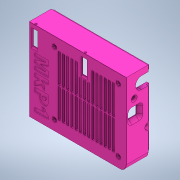
# Autodesk Inventor part: Rambo Case P1.0
Saved by Autodesk Inventor 2020.3 (Build 243373010, 373A)
## iProperties
Created: 2019-12-21
Part Number: Rambo Case P1.0
Material: Generic
Document SubType Name: Modeling
Designer: pepd9
Density: 1 g/cm^3
Appearance: Default
Author: pepd9
Autodesk Inventor part; units mm, degrees
(part 1 of 2)
ref_plane "YZ Plane" through (0, 0, 0) normal (1, 0, 0) x (0, 1, 0)
ref_plane "XZ Plane" through (0, 0, 0) normal (0, 1, 0) x (-1, 0, 0)
ref_plane "Work Plane1" through (0, 0, 3) normal (0, 0, 1) x (1, 0, 0)
sketch "Sketch1" plane through (0, 0, 3) normal (0, 0, 1) x (1, 0, 0)
  circle A0 centre (48.26, 47.625) radius 1.5 construction
  circle A1 centre (48.26, -47.625) radius 1.5 construction
  circle A2 centre (-48.26, -47.625) radius 1.5 construction
  circle A3 centre (-48.26, 47.625) radius 1.5 construction
  line L0 (60.26, 61.625) -> (-86.26, 61.625)
  line L1 (-86.26, 61.625) -> (-86.26, -62.625)
  line L2 (-86.26, -62.625) -> (60.26, -62.625)
  line L3 (60.26, -62.625) -> (60.26, 61.625)
  point P0 (0, 0)
  dimension "d1" = 14
  dimension "d2" = 12
  dimension "d3" = 38
  dimension "d4" = 15
  constraints: 8 end point, 2 parallel, 1 horizontal, 1 perpendicular
  measures "d1" distance from line of L0 A0.centre
  measures "d2" distance from line of L3 A0.centre
  measures "d3" distance from line of L1 A3.centre
  measures "d4" distance from line of L2 A1.centre
extrude "Extrusion1" add sketch "Sketch1" along normal blind 3
sketch "Sketch2" plane through (0, 0, 3) normal (0, 0, -1) x (-1, 0, 0)
  line L0 (-60.26, -62.625) -> (-60.26, 61.625) projected
  line L1 (86.26, -62.625) -> (-60.26, -62.625) projected
  line L2 (86.26, 61.625) -> (86.26, -62.625) projected
  line L3 (-60.26, 61.625) -> (86.26, 61.625) projected
  line L4 (-60.26, -62.625) -> (-60.26, 61.625) projected
  line L5 (86.26, -62.625) -> (-60.26, -62.625) projected
  line L6 (-60.26, 61.625) -> (-54.26, 61.625)
  line L7 (-54.26, 61.625) -> (-54.26, -62.625)
  line L8 (-54.26, -62.625) -> (-60.26, -62.625)
  line L9 (-60.26, -62.625) -> (-60.26, 61.625)
  line L10 (-54.26, -62.625) -> (86.26, -62.625)
  line L11 (86.26, -62.625) -> (86.26, -56.625)
  line L12 (86.26, -56.625) -> (-54.26, -56.625)
  line L13 (-54.26, -56.625) -> (-54.26, -62.625)
  line L14 (86.26, 61.625) -> (86.26, -62.625) projected
  line L15 (-54.26, 61.625) -> (86.26, 61.625)
  line L16 (86.26, 61.625) -> (86.26, 55.625)
  line L17 (86.26, 55.625) -> (-54.26, 55.625)
  line L18 (-54.26, 55.625) -> (-54.26, 61.625)
  point P0 (0, 0)
  dimension "d7" = 6
  dimension "d10" = 6
  dimension "d11" = 6
  constraints: 24 end point, 6 parallel, 3 horizontal, 3 perpendicular, 3 point on line
  measures "d7" distance of L7.end L8.end
  measures "d10" distance of L11.end L10.end
  measures "d11" distance of L15.end L16.end
extrude "Extrusion2" add sketch "Sketch2" along normal blind 30 contours L0 L3 L7 L1 | L7 L12 L2 L1 | L3 L2 L17 L7
sketch "Sketch3" plane through (0, 0, 3) normal (0, 0, -1) x (-1, 0, 0)
  circle A0 centre (-48.26, -47.625) radius 1.5 construction
  circle A1 centre (-48.26, 47.625) radius 1.5 construction
  circle A2 centre (48.26, -47.625) radius 1.5 construction
  circle A3 centre (48.26, 47.625) radius 1.5 construction
  line L0 (-52.26, -45.3156) -> (-48.26, -43.0062)
  line L1 (-48.26, -43.0062) -> (-44.26, -45.3156)
  line L2 (-44.26, -45.3156) -> (-44.26, -49.9344)
  line L3 (-44.26, -49.9344) -> (-48.26, -52.2438)
  line L4 (-48.26, -52.2438) -> (-52.26, -49.9344)
  line L5 (-52.26, -49.9344) -> (-52.26, -45.3156)
  line L6 (-52.26, 49.9344) -> (-48.26, 52.2438)
  line L7 (-48.26, 52.2438) -> (-44.26, 49.9344)
  line L8 (-44.26, 49.9344) -> (-44.26, 45.3156)
  line L9 (-44.26, 45.3156) -> (-48.26, 43.0062)
  line L10 (-48.26, 43.0062) -> (-52.26, 45.3156)
  line L11 (-52.26, 45.3156) -> (-52.26, 49.9344)
  line L12 (44.26, 49.9344) -> (48.26, 52.2438)
  line L13 (48.26, 52.2438) -> (52.26, 49.9344)
  line L14 (52.26, 49.9344) -> (52.26, 45.3156)
  line L15 (52.26, 45.3156) -> (48.26, 43.0062)
  line L16 (48.26, 43.0062) -> (44.26, 45.3156)
  line L17 (44.26, 45.3156) -> (44.26, 49.9344)
  line L18 (44.26, -45.3156) -> (48.26, -43.0062)
  line L19 (48.26, -43.0062) -> (52.26, -45.3156)
  line L20 (52.26, -45.3156) -> (52.26, -49.9344)
  line L21 (52.26, -49.9344) -> (48.26, -52.2438)
  line L22 (48.26, -52.2438) -> (44.26, -49.9344)
  line L23 (44.26, -49.9344) -> (44.26, -45.3156)
  point P0 (0, 0)
  point P1 (44.26, -47.625)
  dimension "d12" = 8
  dimension "d13" = 8
  dimension "d14" = 8
  dimension "d15" = 8
  constraints: 48 end point, 4 coincident, 3 vertical, 1 midpoint, 1 point on line, 52 other
  measures "d12" distance between parallel lines of L20 L23
  measures "d13" distance between parallel lines of L17 L14
  measures "d14" distance between parallel lines of L8 L11
  measures "d15" distance between parallel lines of L5 L2
extrude "Extrusion3" add sketch "Sketch3" along normal blind 4
sketch "Sketch4" plane through (0, 0, -1) normal (0, 0, -1) x (-1, 0, 0)
  circle A0 centre (-48.26, -47.625) radius 1.5 projected
  circle A1 centre (-48.26, 47.625) radius 1.5 projected
  circle A2 centre (48.26, 47.625) radius 1.5 projected
  circle A3 centre (48.26, -47.625) radius 1.5 projected
  point P0 (0, 0)
hole "Hole1" at (48.26, -47.625, -1) at (48.26, 47.625, -1) at (-48.26, 47.625, -1) at (-48.26, -47.625, -1) direction (0, 0, 1) diameter 3.2 end through all clearance for "Socket Head Cap Screw" size "M3" standard "Ansi Metric M Profile"
sketch "Sketch5" plane through (60.26, -62.625, 6) normal (1, 0, 0) x (0, 0, -1)
  arc A0 (8.5, 75.51) -> (8, 75.01) centre (8.5, 75.01) ccw projected
  line L0 (8.5, 75.51) -> (18.7, 75.51) projected
  arc A1 (19.2, 75.01) -> (18.7, 75.51) centre (18.7, 75.01) ccw projected
  line L1 (19.2, 64.21) -> (19.2, 75.01) projected
  arc A2 (18.7, 63.71) -> (19.2, 64.21) centre (18.7, 64.21) ccw projected
  line L2 (8.5, 63.71) -> (18.7, 63.71) projected
  arc A3 (8, 64.21) -> (8.5, 63.71) centre (8.5, 64.21) ccw projected
  line L3 (8, 75.01) -> (8, 64.21) projected
  arc A4 (7.4, 64.21) -> (8.5, 63.11) centre (8.5, 64.21) ccw
  line L4 (8.5, 63.11) -> (18.7, 63.11)
  arc A5 (18.7, 63.11) -> (19.8, 64.21) centre (18.7, 64.21) ccw
  line L5 (19.8, 64.21) -> (19.8, 75.01)
  arc A6 (19.8, 75.01) -> (18.7, 76.11) centre (18.7, 75.01) ccw
  line L6 (18.7, 76.11) -> (8.5, 76.11)
  arc A7 (8.5, 76.11) -> (7.4, 75.01) centre (8.5, 75.01) ccw
  line L7 (7.4, 75.01) -> (7.4, 64.21)
  point P0 (6, 62.625)
  dimension "d25" = 0.6
  constraints: 8 end point, 8 point on circle, 4 centre point, 7 other
  measures "d25" distance between parallel lines of L3 L7
extrude "Extrusion4" cut sketch "Sketch5" against normal up to surface (6 mm away) contours L0 A1 L1 A2 L2 A3 L3 A0 | L7 A7 L6 A6 L5 A5 L4 A4
sketch "Sketch6" plane through (60.26, -62.625, 6) normal (1, 0, 0) x (0, 0, -1)
  circle A0 centre (12, 90.819) radius 1.27
  line L0 (0, 0) -> (0, 124.25) projected
  point P0 (6, 62.625)
  dimension "d106" = 2.54
  dimension "d107" = 12
  constraints: 1 centre point
  measures "d106" diameter of A0
  measures "d107" distance from line of L0 A0.centre
hole "Hole2" at (60.26, 28.194, -6) direction (-1, 0, 0) diameter 5 end through all
chamfer "Chamfer2" distance 2 angle 45 1 edges at (60.26, 28.194, -3.5)
sketch "Sketch7" plane through (-86.26, 55.625, 3) normal (0, -1, 0) x (1, 0, 0)
  circle A0 centre (82.9724, 1) radius 1.1 projected
  circle A1 centre (8.1724, 1) radius 1.1 projected
  circle A2 centre (8.1724, 1) radius 1.1 projected
  point P0 (86.26, -3)
hole "Hole3" at (-3.2876, 55.625, 4) at (-78.0876, 55.625, 4) direction (0, 1, 0) diameter 3.2 end through all clearance for "Socket Head Cap Screw" size "M3" standard "Ansi Metric M Profile"
sketch "Sketch8" plane through (-86.26, 55.625, -27) normal (0, -1, 0) x (1, 0, 0)
  arc A0 (81.7234, 30) -> (84.2214, 30) centre (82.9724, 31) ccw projected
  arc A1 (6.9234, 30) -> (9.4214, 30) centre (8.1724, 31) ccw projected
  point P0 (86.26, 27)
  point P1 (5.1724, 31)
hole "Hole4" at (-3.2876, 55.625, 4) at (-78.0876, 55.625, 4) direction (0, -1, 0) diameter 10 depth 25
sketch "Sketch9" plane through (0, 0, 6) normal (0, 0, 1) x (1, 0, 0)
  line L0 (1.295, 55.625) -> (1.295, 30.625) projected
  line L1 (1.295, 30.625) -> (-7.8702, 30.625) projected
  line L2 (-7.8702, 30.625) -> (-7.8702, 55.625) projected
  line L3 (-7.8702, 55.625) -> (1.295, 55.625) projected
  line L4 (-73.505, 55.625) -> (-73.505, 30.625) projected
  line L5 (-73.505, 30.625) -> (-82.6702, 30.625) projected
  line L6 (-82.6702, 30.625) -> (-82.6702, 55.625) projected
  line L7 (-82.6702, 55.625) -> (-73.505, 55.625) projected
  circle A0 centre (-48.26, 47.625) radius 1.6 projected
  circle A1 centre (48.26, -47.625) radius 1.6 projected
  circle A2 centre (48.26, 47.625) radius 1.6 projected
  circle A3 centre (-48.26, -47.625) radius 1.6 projected
  line L8 (60.26, 61.625) -> (-86.26, 61.625) projected
  line L9 (-86.26, 61.625) -> (-86.26, -62.625) projected
  line L10 (-86.26, -62.625) -> (60.26, -62.625) projected
  line L11 (60.26, -62.625) -> (60.26, 61.625) projected
  line L12 (51.01, 46.0373) -> (48.26, 44.4496)
  line L13 (48.26, 44.4496) -> (45.51, 46.0373)
  line L14 (45.51, 46.0373) -> (45.51, 49.2127)
  line L15 (45.51, 49.2127) -> (48.26, 50.8004)
  line L16 (48.26, 50.8004) -> (51.01, 49.2127)
  line L17 (51.01, 49.2127) -> (51.01, 46.0373)
  line L18 (51.01, -49.2127) -> (48.26, -50.8004)
  line L19 (48.26, -50.8004) -> (45.51, -49.2127)
  line L20 (45.51, -49.2127) -> (45.51, -46.0373)
  line L21 (45.51, -46.0373) -> (48.26, -44.4496)
  line L22 (48.26, -44.4496) -> (51.01, -46.0373)
  line L23 (51.01, -46.0373) -> (51.01, -49.2127)
  circle A4 centre (-48.26, -47.625) radius 1.6 projected
  line L24 (-45.51, -49.2127) -> (-48.26, -50.8004)
  line L25 (-48.26, -50.8004) -> (-51.01, -49.2127)
  line L26 (-51.01, -49.2127) -> (-51.01, -46.0373)
  line L27 (-51.01, -46.0373) -> (-48.26, -44.4496)
  line L28 (-48.26, -44.4496) -> (-45.51, -46.0373)
  line L29 (-45.51, -46.0373) -> (-45.51, -49.2127)
  line L30 (-45.51, 46.0373) -> (-48.26, 44.4496)
  line L31 (-48.26, 44.4496) -> (-51.01, 46.0373)
  line L32 (-51.01, 46.0373) -> (-51.01, 49.2127)
  line L33 (-51.01, 49.2127) -> (-48.26, 50.8004)
  line L34 (-48.26, 50.8004) -> (-45.51, 49.2127)
  line L35 (-45.51, 49.2127) -> (-45.51, 46.0373)
  point P0 (0, 0)
  point P1 (-45.51, 47.625)
  dimension "d55" = 5.5
  dimension "d56" = 5.5
  dimension "d57" = 5.5
  constraints: 48 end point, 4 coincident, 4 vertical, 1 midpoint, 1 point on line, 52 other
  measures "d55" distance between parallel lines of L17 L14
  measures "d56" distance between parallel lines of L20 L23
  measures "d57" distance between parallel lines of L26 L29
extrude "Extrusion5" cut sketch "Sketch9" against normal blind 3 contours L12 L13 L14 L15 L16 L17 | L18 L19 L20 L21 L22 L23 | L24 L25 L26 L27 L28 L29 | L30 L31 L32 L33 L34 L35
sketch "Sketch10" plane through (0, 0, 6) normal (0, 0, 1) x (1, 0, 0)
  line L0 (-4, 45.0147) -> (-1, 45.0147)
  line L1 (-1, 45.0147) -> (-1, -44.9853)
  line L2 (-1, -44.9853) -> (-4, -44.9853)
  line L3 (-4, -44.9853) -> (-4, 45.0147)
  line L4 (-4, 45.0147) -> (-1, -44.9853) construction
  line L5 (-1, 45.0147) -> (-4, -44.9853) construction
  line L6 (45.51, -46.0373) -> (48.26, -44.4496) projected
  line L7 (48.26, -44.4496) -> (51.01, -46.0373) projected
  line L8 (51.01, -46.0373) -> (51.01, -49.2127) projected
  line L9 (51.01, -49.2127) -> (48.26, -50.8004) projected
  line L10 (48.26, -50.8004) -> (45.51, -49.2127) projected
  line L11 (45.51, -49.2127) -> (45.51, -46.0373) projected
  line L12 (-48.26, -50.8004) -> (-51.01, -49.2127) projected
  line L13 (-51.01, -49.2127) -> (-51.01, -46.0373) projected
  line L14 (-51.01, -46.0373) -> (-48.26, -44.4496) projected
  line L15 (-48.26, -44.4496) -> (-45.51, -46.0373) projected
  line L16 (-45.51, -46.0373) -> (-45.51, -49.2127) projected
  line L17 (-45.51, -49.2127) -> (-48.26, -50.8004) projected
  line L18 (48.26, 44.4496) -> (45.51, 46.0373) projected
  line L19 (45.51, 46.0373) -> (45.51, 49.2127) projected
  line L20 (45.51, 49.2127) -> (48.26, 50.8004) projected
  line L21 (48.26, 50.8004) -> (51.01, 49.2127) projected
  line L22 (51.01, 49.2127) -> (51.01, 46.0373) projected
  line L23 (51.01, 46.0373) -> (48.26, 44.4496) projected
  line L24 (-45.51, 49.2127) -> (-45.51, 46.0373) projected
  line L25 (-45.51, 46.0373) -> (-48.26, 44.4496) projected
  line L26 (-48.26, 44.4496) -> (-51.01, 46.0373) projected
  line L27 (-51.01, 46.0373) -> (-51.01, 49.2127) projected
  line L28 (-51.01, 49.2127) -> (-48.26, 50.8004) projected
  line L29 (-48.26, 50.8004) -> (-45.51, 49.2127) projected
  line L30 (1.295, 55.625) -> (1.295, 30.625) projected
  line L31 (1.295, 30.625) -> (-7.8702, 30.625) projected
  line L32 (-7.8702, 30.625) -> (-7.8702, 55.625) projected
  line L33 (-7.8702, 55.625) -> (1.295, 55.625) projected
  line L34 (-73.505, 55.625) -> (-73.505, 30.625) projected
  line L35 (-73.505, 30.625) -> (-82.6702, 30.625) projected
  line L36 (-82.6702, 30.625) -> (-82.6702, 55.625) projected
  line L37 (-82.6702, 55.625) -> (-73.505, 55.625) projected
  line L38 (60.26, 61.625) -> (-86.26, 61.625) projected
  line L39 (-86.26, 61.625) -> (-86.26, -62.625) projected
  line L40 (-86.26, -62.625) -> (60.26, -62.625) projected
  line L41 (60.26, -62.625) -> (60.26, 61.625) projected
  line L42 (5.295, 26.625) -> (5.295, 59.625)
  line L43 (5.295, 59.625) -> (-11.8702, 59.625)
  line L44 (-11.8702, 59.625) -> (-11.8702, 26.625)
  line L45 (-11.8702, 26.625) -> (5.295, 26.625)
  line L46 (2.2, 45.0147) -> (5.2, 45.0147)
  line L47 (2.2, -44.9853) -> (2.2, 45.0147)
  line L48 (5.2, 45.0147) -> (5.2, -44.9853)
  line L49 (5.2, -44.9853) -> (2.2, -44.9853)
  line L50 (8.4, 45.0147) -> (11.4, 45.0147)
  line L51 (8.4, -44.9853) -> (8.4, 45.0147)
  line L52 (11.4, 45.0147) -> (11.4, -44.9853)
  line L53 (11.4, -44.9853) -> (8.4, -44.9853)
  line L54 (14.6, 45.0147) -> (17.6, 45.0147)
  line L55 (14.6, -44.9853) -> (14.6, 45.0147)
  line L56 (17.6, 45.0147) -> (17.6, -44.9853)
  line L57 (17.6, -44.9853) -> (14.6, -44.9853)
  line L58 (20.8, 45.0147) -> (23.8, 45.0147)
  line L59 (20.8, -44.9853) -> (20.8, 45.0147)
  line L60 (23.8, 45.0147) -> (23.8, -44.9853)
  line L61 (23.8, -44.9853) -> (20.8, -44.9853)
  line L62 (27, 45.0147) -> (30, 45.0147)
  line L63 (27, -44.9853) -> (27, 45.0147)
  line L64 (30, 45.0147) -> (30, -44.9853)
  line L65 (30, -44.9853) -> (27, -44.9853)
  line L66 (33.2, 45.0147) -> (36.2, 45.0147)
  line L67 (33.2, -44.9853) -> (33.2, 45.0147)
  line L68 (36.2, 45.0147) -> (36.2, -44.9853)
  line L69 (36.2, -44.9853) -> (33.2, -44.9853)
  line L70 (39.4, 45.0147) -> (42.4, 45.0147)
  line L71 (39.4, -44.9853) -> (39.4, 45.0147)
  line L72 (42.4, 45.0147) -> (42.4, -44.9853)
  line L73 (42.4, -44.9853) -> (39.4, -44.9853)
  line L74 (-10.4, -44.9853) -> (-10.4, 45.0147)
  line L75 (-7.4, 45.0147) -> (-7.4, -44.9853)
  line L76 (-10.4, 45.0147) -> (-7.4, 45.0147)
  line L77 (-7.4, -44.9853) -> (-10.4, -44.9853)
  line L78 (-16.8, -44.9853) -> (-16.8, 45.0147)
  line L79 (-13.8, 45.0147) -> (-13.8, -44.9853)
  line L80 (-16.8, 45.0147) -> (-13.8, 45.0147)
  line L81 (-13.8, -44.9853) -> (-16.8, -44.9853)
  line L82 (-23.2, -44.9853) -> (-23.2, 45.0147)
  line L83 (-20.2, 45.0147) -> (-20.2, -44.9853)
  line L84 (-23.2, 45.0147) -> (-20.2, 45.0147)
  line L85 (-20.2, -44.9853) -> (-23.2, -44.9853)
  line L86 (-29.6, -44.9853) -> (-29.6, 45.0147)
  line L87 (-26.6, 45.0147) -> (-26.6, -44.9853)
  line L88 (-29.6, 45.0147) -> (-26.6, 45.0147)
  line L89 (-26.6, -44.9853) -> (-29.6, -44.9853)
  line L90 (-36, -44.9853) -> (-36, 45.0147)
  line L91 (-33, 45.0147) -> (-33, -44.9853)
  line L92 (-36, 45.0147) -> (-33, 45.0147)
  line L93 (-33, -44.9853) -> (-36, -44.9853)
  line L94 (-42.4, -44.9853) -> (-42.4, 45.0147)
  line L95 (-39.4, 45.0147) -> (-39.4, -44.9853)
  line L96 (-42.4, 45.0147) -> (-39.4, 45.0147)
  line L97 (-39.4, -44.9853) -> (-42.4, -44.9853)
  point P0 (-7.4, 26.625)
  point P1 (-10.4, 26.625)
  point P2 (-1, 26.625)
  point P3 (-4, 26.625)
  point P4 (4.1765, 45.0147)
  point P5 (2.2, 26.625)
  point P6 (5.2, 26.625)
  dimension "d60" = 3
  dimension "d61" = 90
  dimension "d62" = 4
  dimension "d65" = 6.2
  dimension "d72" = 6.4
  dimension "d77" = 3.11
  dimension "d78" = 1.0226
  constraints: 124 end point, 3 horizontal, 2 collinear, 2 parallel, 1 perpendicular, 105 other
  measures "d60" distance of L1.end L2.end
  measures "d61" distance of L0.end L1.end
  measures "d62" distance between parallel lines of L30 L42
  measures "d65" distance of L0.start L46.start
  measures "d72" distance of L2.end L74.start
  measures "d77" distance between parallel lines of L19 L72
  measures "d78" distance from line of L18.end L70
extrude "Extrusion6" cut sketch "Sketch10" against normal blind 3 contours L45 L1 L2 L3 | L75 L77 L74 L45 | L45 L48 L49 L47 | L50 L52 L53 L51 | L54 L56 L57 L55 | L58 L60 L61 L59 | L62 L64 L65 L63 | L66 L68 L69 L67 | L70 L72 L73 L71 | L78 L80 L79 L81 | L82 L84 L83 L85 | L86 L88 L87 L89 | L90 L92 L91 L93 | L94 L96 L95 L97
sketch "Sketch11" plane through (0, 0, 6) normal (0, 0, 1) x (1, 0, 0)
  line L0 (45.51, -46.0373) -> (48.26, -44.4496) projected
  line L1 (48.26, -44.4496) -> (51.01, -46.0373) projected
  line L2 (51.01, -46.0373) -> (51.01, -49.2127) projected
  line L3 (51.01, -49.2127) -> (48.26, -50.8004) projected
  line L4 (48.26, -50.8004) -> (45.51, -49.2127) projected
  line L5 (45.51, -49.2127) -> (45.51, -46.0373) projected
  line L6 (-48.26, -50.8004) -> (-51.01, -49.2127) projected
  line L7 (-51.01, -49.2127) -> (-51.01, -46.0373) projected
  line L8 (-51.01, -46.0373) -> (-48.26, -44.4496) projected
  line L9 (-48.26, -44.4496) -> (-45.51, -46.0373) projected
  line L10 (-45.51, -46.0373) -> (-45.51, -49.2127) projected
  line L11 (-45.51, -49.2127) -> (-48.26, -50.8004) projected
  line L12 (48.26, 44.4496) -> (45.51, 46.0373) projected
  line L13 (45.51, 46.0373) -> (45.51, 49.2127) projected
  line L14 (45.51, 49.2127) -> (48.26, 50.8004) projected
  line L15 (48.26, 50.8004) -> (51.01, 49.2127) projected
  line L16 (51.01, 49.2127) -> (51.01, 46.0373) projected
  line L17 (51.01, 46.0373) -> (48.26, 44.4496) projected
  line L18 (-45.51, 49.2127) -> (-45.51, 46.0373) projected
  line L19 (-45.51, 46.0373) -> (-48.26, 44.4496) projected
  line L20 (-48.26, 44.4496) -> (-51.01, 46.0373) projected
  line L21 (-51.01, 46.0373) -> (-51.01, 49.2127) projected
  line L22 (-51.01, 49.2127) -> (-48.26, 50.8004) projected
  line L23 (-48.26, 50.8004) -> (-45.51, 49.2127) projected
  line L24 (1.295, 55.625) -> (1.295, 30.625) projected
  line L25 (1.295, 30.625) -> (-7.8702, 30.625) projected
  line L26 (-7.8702, 30.625) -> (-7.8702, 55.625) projected
  line L27 (-7.8702, 55.625) -> (1.295, 55.625) projected
  line L28 (-73.505, 55.625) -> (-73.505, 30.625) projected
  line L29 (-73.505, 30.625) -> (-82.6702, 30.625) projected
  line L30 (-82.6702, 30.625) -> (-82.6702, 55.625) projected
  line L31 (-82.6702, 55.625) -> (-73.505, 55.625) projected
  line L32 (60.26, 61.625) -> (-86.26, 61.625) projected
  line L33 (-86.26, 61.625) -> (-86.26, -62.625) projected
  line L34 (-86.26, -62.625) -> (60.26, -62.625) projected
  line L35 (60.26, -62.625) -> (60.26, 61.625) projected
  line L36 (-42.4, 45.0147) -> (-42.4, -44.9853) projected
  line L37 (42.4, 1.2) -> (-42.4, 1.2)
  line L38 (-42.4, 1.2) -> (-42.4, -1.2)
  line L39 (-42.4, -1.2) -> (42.4, -1.2)
  line L40 (42.4, -1.2) -> (42.4, 1.2)
  line L41 (42.4, 1.2) -> (-42.4, -1.2) construction
  line L42 (-42.4, 1.2) -> (42.4, -1.2) construction
  point P0 (0, 0)
  dimension "d81" = 2.4
  constraints: 12 end point, 2 midpoint, 2 parallel, 1 horizontal, 1 perpendicular, 1 point on line
  measures "d81" distance of L38.end L37.end
extrude "Extrusion7" add sketch "Sketch11" against normal up to surface (3 mm away) contours L37 L40 L39 L36
fillet "Fillet1" radius 0.4 50 edges at (42.4, 45.0147, 4.5) (39.4, 45.0147, 4.5) (36.2, 45.0147, 4.5) (33.2, 45.0147, 4.5) (30, 45.0147, 4.5) (27, 45.0147, 4.5) (23.8, 45.0147, 4.5) (20.8, 45.0147, 4.5) (14.6, 45.0147, 4.5) (17.6, 45.0147, 4.5) (11.4, 45.0147, 4.5) (8.4, 45.0147, 4.5) (42.4, 1.2, 4.5) (39.4, 1.2, 4.5) (39.4, -1.2, 4.5) (42.4, -1.2, 4.5) (42.4, -44.9853, 4.5) (39.4, -44.9853, 4.5) (36.2, -44.9853, 4.5) (33.2, -44.9853, 4.5) (30, -44.9853, 4.5) (27, -44.9853, 4.5) (23.8, -44.9853, 4.5) (20.8, -44.9853, 4.5) (17.6, -44.9853, 4.5) (14.6, -44.9853, 4.5) (11.4, -44.9853, 4.5) (8.4, -44.9853, 4.5) (5.2, -44.9853, 4.5) (2.2, -44.9853, 4.5) (-1, -44.9853, 4.5) (-4, -44.9853, 4.5) (-7.4, -44.9853, 4.5) (-10.4, -44.9853, 4.5) (-13.8, -44.9853, 4.5) (-16.8, -44.9853, 4.5) (-20.2, -44.9853, 4.5) (-23.2, -44.9853, 4.5) (-26.6, -44.9853, 4.5) (-29.6, -44.9853, 4.5) (-36, -44.9853, 4.5) (-33, -44.9853, 4.5) (-39.4, -44.9853, 4.5) (-42.4, -44.9853, 4.5) (-42.4, -1.2, 4.5) (-42.4, 1.2, 4.5) (-39.4, -1.2, 4.5) (-39.4, 1.2, 4.5) (-36, -1.2, 4.5) (-36, 1.2, 4.5)
fillet "Fillet2" radius 0.4 48 edges at (-33, -1.2, 4.5) (-33, 1.2, 4.5) (-29.6, -1.2, 4.5) (-29.6, 1.2, 4.5) (-26.6, 1.2, 4.5) (-26.6, -1.2, 4.5) (-23.2, -1.2, 4.5) (-23.2, 1.2, 4.5) (-20.2, 1.2, 4.5) (-20.2, -1.2, 4.5) (-16.8, 1.2, 4.5) (-16.8, -1.2, 4.5) (-13.8, 1.2, 4.5) (-13.8, -1.2, 4.5) (-10.4, 1.2, 4.5) (-10.4, -1.2, 4.5) (-7.4, 1.2, 4.5) (-7.4, -1.2, 4.5) (-4, 1.2, 4.5) (-4, -1.2, 4.5) (-1, 1.2, 4.5) (-1, -1.2, 4.5) (2.2, 1.2, 4.5) (2.2, -1.2, 4.5) (5.2, 1.2, 4.5) (5.2, -1.2, 4.5) (8.4, 1.2, 4.5) (8.4, -1.2, 4.5) (11.4, 1.2, 4.5) (11.4, -1.2, 4.5) (14.6, 1.2, 4.5) (14.6, -1.2, 4.5) (17.6, -1.2, 4.5) (17.6, 1.2, 4.5) (20.8, -1.2, 4.5) (23.8, -1.2, 4.5) (20.8, 1.2, 4.5) (23.8, 1.2, 4.5) (27, -1.2, 4.5) (27, 1.2, 4.5) (30, 1.2, 4.5) (30, -1.2, 4.5) (33.2, -1.2, 4.5) (36.2, -1.2, 4.5) (36.2, 1.2, 4.5) (33.2, 1.2, 4.5) (5.2, 26.625, 4.5) (2.2, 26.625, 4.5)
fillet "Fillet3" radius 0.4 14 edges at (-1, 26.625, 4.5) (-4, 26.625, 4.5) (-7.4, 26.625, 4.5) (-10.4, 26.625, 4.5) (-13.8, 45.0147, 4.5) (-16.8, 45.0147, 4.5) (-20.2, 45.0147, 4.5) (-23.2, 45.0147, 4.5) (-26.6, 45.0147, 4.5) (-29.6, 45.0147, 4.5) (-33, 45.0147, 4.5) (-36, 45.0147, 4.5) (-39.4, 45.0147, 4.5) (-42.4, 45.0147, 4.5)
sketch "Sketch12" plane through (0, 0, 3) normal (0, 0, 1) x (1, 0, 0)
  line L0 (45.51, 46.0373) -> (45.51, 49.2127) projected
  line L1 (48.26, 44.4496) -> (45.51, 46.0373) projected
  line L2 (51.01, 46.0373) -> (48.26, 44.4496) projected
  line L3 (51.01, 49.2127) -> (51.01, 46.0373) projected
  line L4 (48.26, 50.8004) -> (51.01, 49.2127) projected
  line L5 (45.51, 49.2127) -> (48.26, 50.8004) projected
  circle A0 centre (48.26, 47.625) radius 1.6 projected
  line L6 (48.26, -44.4496) -> (51.01, -46.0373) projected
  line L7 (45.51, -46.0373) -> (48.26, -44.4496) projected
  line L8 (45.51, -49.2127) -> (45.51, -46.0373) projected
  line L9 (48.26, -50.8004) -> (45.51, -49.2127) projected
  line L10 (51.01, -49.2127) -> (48.26, -50.8004) projected
  line L11 (51.01, -46.0373) -> (51.01, -49.2127) projected
  circle A1 centre (48.26, -47.625) radius 1.6 projected
  circle A2 centre (-48.26, -47.625) radius 1.6 projected
  line L12 (-51.01, -49.2127) -> (-51.01, -46.0373) projected
  line L13 (-48.26, -50.8004) -> (-51.01, -49.2127) projected
  line L14 (-45.51, -49.2127) -> (-48.26, -50.8004) projected
  line L15 (-45.51, -46.0373) -> (-45.51, -49.2127) projected
  line L16 (-48.26, -44.4496) -> (-45.51, -46.0373) projected
  line L17 (-51.01, -46.0373) -> (-48.26, -44.4496) projected
  circle A3 centre (-48.26, -47.625) radius 1.6 projected
  line L18 (-45.51, 46.0373) -> (-48.26, 44.4496) projected
  line L19 (-45.51, 49.2127) -> (-45.51, 46.0373) projected
  line L20 (-48.26, 50.8004) -> (-45.51, 49.2127) projected
  line L21 (-51.01, 49.2127) -> (-48.26, 50.8004) projected
  line L22 (-51.01, 46.0373) -> (-51.01, 49.2127) projected
  line L23 (-48.26, 44.4496) -> (-51.01, 46.0373) projected
  circle A4 centre (-48.26, 47.625) radius 1.6 projected
  line L24 (-51.6643, -46.025) -> (-44.8557, -46.025)
  line L25 (-44.8557, -46.025) -> (-44.8557, -49.225)
  line L26 (-44.8557, -49.225) -> (-51.6643, -49.225)
  line L27 (-51.6643, -49.225) -> (-51.6643, -46.025)
  line L28 (-51.6643, -46.025) -> (-44.8557, -49.225) construction
  line L29 (-44.8557, -46.025) -> (-51.6643, -49.225) construction
  line L30 (-52.2121, 49.2127) -> (-44.3079, 49.2127)
  line L31 (-44.3079, 49.2127) -> (-44.3079, 46.0373)
  line L32 (-44.3079, 46.0373) -> (-52.2121, 46.0373)
  line L33 (-52.2121, 46.0373) -> (-52.2121, 49.2127)
  line L34 (-52.2121, 49.2127) -> (-44.3079, 46.0373) construction
  line L35 (-44.3079, 49.2127) -> (-52.2121, 46.0373) construction
  line L36 (44.4974, 49.2127) -> (52.0226, 49.2127)
  line L37 (52.0226, 49.2127) -> (52.0226, 46.0373)
  line L38 (52.0226, 46.0373) -> (44.4974, 46.0373)
  line L39 (44.4974, 46.0373) -> (44.4974, 49.2127)
  circle A5 centre (48.26, 47.625) radius 1.6 projected
  line L40 (44.4974, 49.2127) -> (52.0226, 46.0373) construction
  line L41 (52.0226, 49.2127) -> (44.4974, 46.0373) construction
  line L42 (44.7504, -46.025) -> (51.7696, -46.025)
  line L43 (51.7696, -46.025) -> (51.7696, -49.225)
  line L44 (51.7696, -49.225) -> (44.7504, -49.225)
  line L45 (44.7504, -49.225) -> (44.7504, -46.025)
  line L46 (44.7504, -46.025) -> (51.7696, -49.225) construction
  line L47 (51.7696, -46.025) -> (44.7504, -49.225) construction
  point P0 (0, 0)
  point P1 (-45.5313, -46.025)
  point P2 (-48.26, -46.025)
  point P3 (-48.26, -49.225)
  point P4 (-45.5313, -49.225)
  point P5 (-50.9887, -49.225)
  point P6 (-50.9887, -46.025)
  point P7 (-48.0621, 46.0373)
  point P8 (-48.0621, 49.2127)
  point P9 (-48.4579, 46.0373)
  point P10 (-48.4579, 49.2127)
  point P11 (48.4579, 46.0373)
  point P12 (48.4579, 49.2127)
  point P13 (48.0621, 46.0373)
  point P14 (48.0621, 49.2127)
  point P15 (45.5313, -49.225)
  point P16 (48.26, -49.225)
  point P17 (48.26, -46.025)
  point P18 (45.5313, -46.025)
  point P19 (50.9887, -46.025)
  point P20 (50.9887, -49.225)
  constraints: 48 end point, 8 midpoint, 8 parallel, 4 horizontal, 4 perpendicular, 2 point on line
extrude "Extrusion8" cut sketch "Sketch12" against normal blind 0.5 contours L0 L36 A0 L38 | L38 A0 L36 L3 | L6 L11 L10 L44 A1 L42 | L42 A1 L44 L9 L8 L7 | A2 L24 L16 L15 L14 L26 | A2 L26 L13 L12 L17 L24 | L32 A4 L30 L19 | L22 L30 A4 L32
sketch "Sketch13" plane through (0, 0, 2.5) normal (0, 0, 1) x (1, 0, 0)
  line L0 (-48.26, -49.225) -> (-50.9887, -49.225) projected
  arc A0 (-48.26, -46.025) -> (-48.26, -49.225) centre (-48.26, -47.625) ccw projected
  line L1 (-50.9887, -46.025) -> (-48.26, -46.025) projected
  line L2 (-51.01, -46.0373) -> (-50.9887, -46.025) projected
  line L3 (-51.01, -49.2127) -> (-51.01, -46.0373) projected
  line L4 (-50.9887, -49.225) -> (-51.01, -49.2127) projected
  line L5 (-48.26, -46.025) -> (-45.5313, -46.025) projected
  arc A1 (-48.26, -49.225) -> (-48.26, -46.025) centre (-48.26, -47.625) ccw projected
  line L6 (-45.5313, -49.225) -> (-48.26, -49.225) projected
  line L7 (-45.51, -49.2127) -> (-45.5313, -49.225) projected
  line L8 (-45.51, -46.0373) -> (-45.51, -49.2127) projected
  line L9 (-45.5313, -46.025) -> (-45.51, -46.0373) projected
  line L10 (-49.86, -43.9294) -> (-46.66, -43.9294)
  line L11 (-46.66, -43.9294) -> (-46.66, -51.3206)
  line L12 (-46.66, -51.3206) -> (-49.86, -51.3206)
  line L13 (-49.86, -51.3206) -> (-49.86, -43.9294)
  line L14 (-49.86, -43.9294) -> (-46.66, -51.3206) construction
  line L15 (-46.66, -43.9294) -> (-49.86, -51.3206) construction
  line L16 (-45.51, 46.0373) -> (-48.0621, 46.0373) projected
  line L17 (-45.51, 49.2127) -> (-45.51, 46.0373) projected
  line L18 (-48.0621, 49.2127) -> (-45.51, 49.2127) projected
  arc A2 (-48.0621, 46.0373) -> (-48.0621, 49.2127) centre (-48.26, 47.625) ccw projected
  arc A3 (-48.4579, 49.2127) -> (-48.4579, 46.0373) centre (-48.26, 47.625) ccw projected
  line L19 (-51.01, 49.2127) -> (-48.4579, 49.2127) projected
  line L20 (-51.01, 46.0373) -> (-51.01, 49.2127) projected
  line L21 (-48.4579, 46.0373) -> (-51.01, 46.0373) projected
  arc A4 (48.0621, 49.2127) -> (48.0621, 46.0373) centre (48.26, 47.625) ccw projected
  line L22 (45.51, 49.2127) -> (48.0621, 49.2127) projected
  line L23 (45.51, 46.0373) -> (45.51, 49.2127) projected
  line L24 (48.0621, 46.0373) -> (45.51, 46.0373) projected
  line L25 (51.01, 49.2127) -> (51.01, 46.0373) projected
  line L26 (48.4579, 49.2127) -> (51.01, 49.2127) projected
  arc A5 (48.4579, 46.0373) -> (48.4579, 49.2127) centre (48.26, 47.625) ccw projected
  line L27 (51.01, 46.0373) -> (48.4579, 46.0373) projected
  line L28 (45.5313, -49.225) -> (45.51, -49.2127) projected
  line L29 (48.26, -49.225) -> (45.5313, -49.225) projected
  arc A6 (48.26, -46.025) -> (48.26, -49.225) centre (48.26, -47.625) ccw projected
  line L30 (45.5313, -46.025) -> (48.26, -46.025) projected
  line L31 (45.51, -46.0373) -> (45.5313, -46.025) projected
  line L32 (45.51, -49.2127) -> (45.51, -46.0373) projected
  line L33 (50.9887, -46.025) -> (51.01, -46.0373) projected
  line L34 (48.26, -46.025) -> (50.9887, -46.025) projected
  arc A7 (48.26, -49.225) -> (48.26, -46.025) centre (48.26, -47.625) ccw projected
  line L35 (50.9887, -49.225) -> (48.26, -49.225) projected
  line L36 (51.01, -49.2127) -> (50.9887, -49.225) projected
  line L37 (51.01, -46.0373) -> (51.01, -49.2127) projected
  line L38 (46.66, -44.2858) -> (49.86, -44.2858)
  line L39 (49.86, -44.2858) -> (49.86, -50.9642)
  line L40 (49.86, -50.9642) -> (46.66, -50.9642)
  line L41 (46.66, -50.9642) -> (46.66, -44.2858)
  circle A8 centre (48.26, -47.625) radius 1.6 projected
  line L42 (46.66, -44.2858) -> (49.86, -50.9642) construction
  line L43 (49.86, -44.2858) -> (46.66, -50.9642) construction
  line L44 (46.66, 51.2284) -> (49.86, 51.2284)
  line L45 (49.86, 51.2284) -> (49.86, 44.0216)
  line L46 (49.86, 44.0216) -> (46.66, 44.0216)
  line L47 (46.66, 44.0216) -> (46.66, 51.2284)
  line L48 (46.66, 51.2284) -> (49.86, 44.0216) construction
  line L49 (49.86, 51.2284) -> (46.66, 44.0216) construction
  line L50 (-49.86, 51.2284) -> (-46.66, 51.2284)
  line L51 (-46.66, 51.2284) -> (-46.66, 44.0216)
  line L52 (-46.66, 44.0216) -> (-49.86, 44.0216)
  line L53 (-49.86, 44.0216) -> (-49.86, 51.2284)
  line L54 (-49.86, 51.2284) -> (-46.66, 44.0216) construction
  line L55 (-46.66, 51.2284) -> (-49.86, 44.0216) construction
  point P0 (0, 0)
  point P1 (49.86, 47.625)
  point P2 (49.86, 49.2127)
  point P3 (49.86, 46.0373)
  point P4 (46.66, 47.625)
  point P5 (46.66, 46.0373)
  point P6 (46.66, 49.2127)
  point P7 (49.86, -49.225)
  point P8 (49.86, -47.625)
  point P9 (49.86, -46.025)
  point P10 (46.66, -46.025)
  point P11 (46.66, -47.625)
  point P12 (46.66, -49.225)
  point P13 (-46.66, -49.225)
  point P14 (-46.66, -47.625)
  point P15 (-46.66, -46.025)
  point P16 (-49.86, -46.025)
  point P17 (-49.86, -47.625)
  point P18 (-49.86, -49.225)
  point P19 (-49.86, 47.625)
  point P20 (-49.86, 46.0373)
  point P21 (-49.86, 49.2127)
  point P22 (-46.66, 47.625)
  point P23 (-46.66, 49.2127)
  point P24 (-46.66, 46.0373)
  constraints: 48 end point, 8 midpoint, 8 parallel, 4 horizontal, 4 perpendicular, 2 point on line
extrude "Extrusion9" cut sketch "Sketch13" against normal blind 0.5 contours L0 L13 A0 | A1 L11 L6 | L13 L1 A0 | A1 L5 L11 | L16 A2 L51 | A2 L18 L51 | L53 A3 L21 | L53 L19 A3 | A4 L47 L22 | A4 L24 L47 | L45 A5 L26 | L27 A5 L45 | L41 A6 L29 | A7 L39 L35 | L41 L30 A6 | A7 L34 L39
fillet "Fillet4" radius 5 1 edges at (54.26, -56.625, -12)
fillet "Fillet4" radius 10 1 edges at (60.26, -62.625, -10.5)
sketch "Sketch14" plane through (0, 0, 3) normal (0, 0, -1) x (-1, 0, 0)
  line L0 (52.26, -45.3156) -> (52.26, -49.9344) projected
  line L1 (52.26, -49.9344) -> (48.26, -52.2438) projected
  line L2 (48.26, -52.2438) -> (44.26, -49.9344) projected
  line L3 (44.26, -49.9344) -> (44.26, -45.3156) projected
  line L4 (44.26, -45.3156) -> (48.26, -43.0062) projected
  line L5 (48.26, -43.0062) -> (52.26, -45.3156) projected
  line L6 (52.26, 45.3156) -> (48.26, 43.0062) projected
  line L7 (48.26, 43.0062) -> (44.26, 45.3156) projected
  line L8 (44.26, 45.3156) -> (44.26, 49.9344) projected
  line L9 (44.26, 49.9344) -> (48.26, 52.2438) projected
  line L10 (48.26, 52.2438) -> (52.26, 49.9344) projected
  line L11 (52.26, 49.9344) -> (52.26, 45.3156) projected
  line L12 (-52.26, -49.9344) -> (-52.26, -45.3156) projected
  line L13 (-52.26, -45.3156) -> (-48.26, -43.0062) projected
  line L14 (-48.26, -43.0062) -> (-44.26, -45.3156) projected
  line L15 (-44.26, -45.3156) -> (-44.26, -49.9344) projected
  line L16 (-44.26, -49.9344) -> (-48.26, -52.2438) projected
  line L17 (-48.26, -52.2438) -> (-52.26, -49.9344) projected
  line L18 (-52.26, 45.3156) -> (-52.26, 49.9344) projected
  line L19 (-52.26, 49.9344) -> (-48.26, 52.2438) projected
  line L20 (-48.26, 52.2438) -> (-44.26, 49.9344) projected
  line L21 (-44.26, 49.9344) -> (-44.26, 45.3156) projected
  line L22 (-44.26, 45.3156) -> (-48.26, 43.0062) projected
  line L23 (-48.26, 43.0062) -> (-52.26, 45.3156) projected
  arc A0 (-54.26, -51.625) -> (-49.26, -56.625) centre (-49.26, -51.625) ccw projected
  line L24 (-49.26, -56.625) -> (86.26, -56.625) projected
  line L25 (86.26, 55.625) -> (86.26, -56.625) projected
  line L26 (86.26, 55.625) -> (82.9866, 55.625) projected
  line L27 (82.9866, 55.625) -> (82.9866, 30.625) projected
  line L28 (82.9866, 30.625) -> (73.1886, 30.625) projected
  line L29 (73.1886, 30.625) -> (73.1886, 55.625) projected
  line L30 (73.1886, 55.625) -> (8.1866, 55.625) projected
  line L31 (8.1866, 55.625) -> (8.1866, 30.625) projected
  line L32 (8.1866, 30.625) -> (-1.6114, 30.625) projected
  line L33 (-1.6114, 30.625) -> (-1.6114, 55.625) projected
  line L34 (-1.6114, 55.625) -> (-54.26, 55.625) projected
  line L35 (-54.26, 55.625) -> (-54.26, -51.625) projected
  circle A1 centre (-48.26, -47.625) radius 1.6 projected
  circle A2 centre (-48.26, 47.625) radius 1.6 projected
  line L36 (-46.26, -56.625) -> (-50.26, -56.625)
  line L37 (-50.26, -56.625) -> (-50.26, 55.625)
  line L38 (-50.26, 55.625) -> (-46.26, 55.625)
  line L39 (-46.26, 55.625) -> (-46.26, -56.625)
  point P0 (0, 0)
  point P1 (-46.26, 51.0891)
  point P2 (-50.26, 51.0891)
  point P3 (-46.26, -51.0891)
  point P4 (-50.26, -51.0891)
  point P5 (-50.26, -56.524)
  point P6 (-46.26, -44.1609)
  point P7 (-46.26, 44.1609)
  point P8 (-50.26, 44.1609)
  point P9 (-50.26, -44.1609)
  dimension "d93" = 2
  dimension "d94" = 2
  constraints: 8 end point, 2 parallel, 2 point on line, 1 horizontal, 1 perpendicular
  measures "d93" distance from line of L37 A1.centre
  measures "d94" distance from line of A1.centre L39
extrude "Extrusion10" add sketch "Sketch14" along normal blind 2 contours L17 L16 L39 L24 A0 L37 | L37 L23 L22 L39 L14 L13 | L37 L34 L39 L20 L19
sketch "Sketch15" plane through (0, 0, 3) normal (0, 0, -1) x (-1, 0, 0)
  line L0 (-46.26, 55.625) -> (-46.26, 51.0891) projected
  line L1 (-46.26, 51.0891) -> (-44.26, 49.9344) projected
  line L2 (-44.26, 49.9344) -> (-44.26, 45.3156) projected
  line L3 (-44.26, 45.3156) -> (-46.26, 44.1609) projected
  line L4 (-46.26, 44.1609) -> (-46.26, -44.1609) projected
  line L5 (-46.26, -44.1609) -> (-44.26, -45.3156) projected
  line L6 (-44.26, -45.3156) -> (-44.26, -49.9344) projected
  line L7 (-44.26, -49.9344) -> (-46.26, -51.0891) projected
  line L8 (-46.26, -51.0891) -> (-46.26, -56.625) projected
  line L9 (-46.26, -56.625) -> (86.26, -56.625) projected
  line L10 (86.26, 55.625) -> (86.26, -56.625) projected
  line L11 (86.26, 55.625) -> (82.9866, 55.625) projected
  line L12 (82.9866, 55.625) -> (82.9866, 30.625) projected
  line L13 (82.9866, 30.625) -> (73.1886, 30.625) projected
  line L14 (73.1886, 30.625) -> (73.1886, 55.625) projected
  line L15 (73.1886, 55.625) -> (8.1866, 55.625) projected
  line L16 (8.1866, 55.625) -> (8.1866, 30.625) projected
  line L17 (8.1866, 30.625) -> (-1.6114, 30.625) projected
  line L18 (-1.6114, 30.625) -> (-1.6114, 55.625) projected
  line L19 (-1.6114, 55.625) -> (-46.26, 55.625) projected
  line L20 (52.26, -45.3156) -> (52.26, -49.9344) projected
  line L21 (52.26, -49.9344) -> (48.26, -52.2438) projected
  line L22 (48.26, -52.2438) -> (44.26, -49.9344) projected
  line L23 (44.26, -49.9344) -> (44.26, -45.3156) projected
  line L24 (44.26, -45.3156) -> (48.26, -43.0062) projected
  line L25 (48.26, -43.0062) -> (52.26, -45.3156) projected
  line L26 (52.26, 45.3156) -> (48.26, 43.0062) projected
  line L27 (48.26, 43.0062) -> (44.26, 45.3156) projected
  line L28 (44.26, 45.3156) -> (44.26, 49.9344) projected
  line L29 (44.26, 49.9344) -> (48.26, 52.2438) projected
  line L30 (48.26, 52.2438) -> (52.26, 49.9344) projected
  line L31 (52.26, 49.9344) -> (52.26, 45.3156) projected
  circle A0 centre (48.26, -47.625) radius 1.6 projected
  line L32 (45.51, 49.2127) -> (45.51, 46.0373) projected
  line L33 (86.26, -56.625) -> (-49.26, -56.625) projected
  line L34 (50.26, -56.625) -> (46.26, -56.625)
  line L35 (46.26, -56.625) -> (46.26, 55.625)
  line L36 (46.26, 55.625) -> (50.26, 55.625)
  line L37 (50.26, 55.625) -> (50.26, -56.625)
  point P0 (0, 0)
  point P1 (50.26, 51.0891)
  point P2 (46.26, 51.0891)
  point P3 (50.26, -44.1609)
  point P4 (50.26, 44.1609)
  point P5 (46.26, 44.1609)
  point P6 (46.26, -44.1609)
  point P7 (50.26, -51.0891)
  point P8 (46.26, -51.0891)
  dimension "d97" = 2
  dimension "d98" = 2
  constraints: 8 end point, 2 parallel, 2 point on line, 1 horizontal, 1 perpendicular
  measures "d97" distance from line of L35 A0.centre
  measures "d98" distance from line of A0.centre L37
extrude "Extrusion11" add sketch "Sketch15" along normal blind 2 contours L15 L37 L30 L29 L35 | L27 L26 L37 L25 L24 L35 | L22 L21 L37 L9 L35
sketch "Sketch16" plane through (60.26, 61.625, 6) normal (1, 0, 0) x (0, 0, -1)
  line L0 (3, -113.25) -> (33, -113.25) projected
  line L1 (3, -6) -> (3, -113.25) projected
  line L2 (3, -6) -> (33, -6) projected
  line L3 (33, -113.25) -> (33, -6) projected
  circle A0 centre (12, -33.431) radius 2.5 projected
  arc A1 (18.7, -61.14) -> (19.8, -60.04) centre (18.7, -60.04) ccw projected
  line L4 (19.8, -60.04) -> (19.8, -49.24) projected
  arc A2 (19.8, -49.24) -> (18.7, -48.14) centre (18.7, -49.24) ccw projected
  line L5 (18.7, -48.14) -> (8.5, -48.14) projected
  arc A3 (8.5, -48.14) -> (7.4, -49.24) centre (8.5, -49.24) ccw projected
  line L6 (7.4, -49.24) -> (7.4, -60.04) projected
  arc A4 (7.4, -60.04) -> (8.5, -61.14) centre (8.5, -60.04) ccw projected
  line L7 (8.5, -61.14) -> (18.7, -61.14) projected
  circle A5 centre (23, -18) radius 9
  line L8 (23, -9) -> (42.1674, -9)
  line L9 (42.1674, -9) -> (42.1674, -27)
  line L10 (42.1674, -27) -> (23, -27)
  line L11 (23, -27) -> (23, -9)
  point P0 (6, -61.625)
  point P1 (23, -27)
  point P2 (33, -27)
  point P3 (33, -9)
  dimension "d101" = 18
  dimension "d102" = 12
  dimension "d103" = 20
  dimension "d114" = 18
  constraints: 8 end point, 2 parallel, 1 horizontal, 1 perpendicular, 3 other
  measures "d102" distance from line of L2 point (23, -18)
  measures "d103" distance from line of L1 point (23, -18)
  measures "d114" distance of L8.end L9.end
extrude "Extrusion12" cut sketch "Sketch16" against normal up to surface (6 mm away) contours L10 A5 L8 L3 | L11 A5 | A5 L11
move faces "Move1" translate (0, 0, -0.5) faces at (58.26, 8.785, -13.8) (56.26, 12.7869, -13.724) (58.26, 0.4881, -12.7822)
chamfer "Chamfer3" distance 5 angle 45 8 edges at (60.26, 13.485, -7.85) (60.26, 13.1628, -13.9778) (60.26, 6.985, -14.3) (60.26, 0.8072, -13.9778) (60.26, 0.485, -7.85) (60.26, 0.8072, -1.7222) (60.26, 6.985, -1.4) (60.26, 13.1628, -1.7222)
sketch "Sketch17" plane through (0, 0, 6) normal (0, 0, 1) x (1, 0, 0)
  line L0 (-57.314, 27.2505) -> (-57.314, -14.6937) construction
  line L1 (-57.314, -14.6937) -> (-66.8026, -14.6937) construction
  line L2 (-66.8026, -14.6937) -> (-66.8026, 27.2505) construction
  line L3 (-66.8026, 27.2505) -> (-57.314, 27.2505) construction
  line L4 (-57.6605, 25.2678) -> (-57.6605, 17.1254)
  line L5 (-57.6605, 17.1254) -> (-69.826, 14.007)
  line L6 (-69.826, 14.007) -> (-57.6605, 10.9079)
  line L7 (-57.6605, 10.9079) -> (-57.6605, 2.7847)
  line L8 (-57.6605, 2.7847) -> (-77.6605, 2.7847)
  line L9 (-77.6605, 2.7847) -> (-77.6605, 7.8472)
  line L10 (-77.6605, 7.8472) -> (-62.3958, 7.8472)
  line L11 (-62.3958, 7.8472) -> (-77.6605, 11.7356)
  line L12 (-77.6605, 11.7356) -> (-77.6605, 16.3169)
  line L13 (-77.6605, 16.3169) -> (-62.3958, 20.2053)
  line L14 (-62.3958, 20.2053) -> (-77.6605, 20.2053)
  line L15 (-77.6605, 20.2053) -> (-77.6605, 25.2678)
  line L16 (-77.6605, 25.2678) -> (-57.6605, 25.2678)
  line L17 (-57.6605, -0.8149) -> (-57.6605, -6.4935)
  line L18 (-57.6605, -6.4935) -> (-67.9588, -6.4935)
  line L19 (-67.9588, -6.4935) -> (-63.1658, -10.6321)
  line L20 (-63.1658, -10.6321) -> (-63.1658, -17.4656)
  line L21 (-63.1658, -17.4656) -> (-68.2476, -12.2683)
  line L22 (-68.2476, -12.2683) -> (-77.6605, -17.7736)
  line L23 (-77.6605, -17.7736) -> (-77.6605, -11.5175)
  line L24 (-77.6605, -11.5175) -> (-71.8664, -8.5724)
  line L25 (-71.8664, -8.5724) -> (-73.8876, -6.4935)
  line L26 (-73.8876, -6.4935) -> (-77.6605, -6.4935)
  line L27 (-77.6605, -6.4935) -> (-77.6605, -0.8149)
  line L28 (-77.6605, -0.8149) -> (-57.6605, -0.8149)
  line L29 (-57.6605, -19.814) -> (-57.6605, -30.0931)
  spline S0 degree 2 poles (-57.6605, -30.0931) (-57.6605, -33.4425) (-60.8558, -36.7919) (-63.801, -36.7919) knots 0 0 0 1 2 2 2
  spline S1 degree 2 poles (-63.801, -36.7919) (-66.8424, -36.7919) (-70.2495, -33.1537) (-70.2495, -29.4194) knots 0 0 0 1 2 2 2
  line L30 (-70.2495, -29.4194) -> (-70.2495, -26.0315)
  line L31 (-70.2495, -26.0315) -> (-77.6605, -26.0315)
  line L32 (-77.6605, -26.0315) -> (-77.6605, -19.814)
  line L33 (-77.6605, -19.814) -> (-57.6605, -19.814)
  line L34 (-66.1879, -26.0315) -> (-66.1879, -27.5329)
  spline S2 degree 2 poles (-66.1879, -27.5329) (-66.1879, -29.3231) (-64.9367, -30.7668) (-63.9742, -30.7668) knots 0 0 0 1 2 2 2
  spline S3 degree 2 poles (-63.9742, -30.7668) (-63.031, -30.7668) (-61.7221, -29.5156) (-61.7221, -27.7832) knots 0 0 0 1 2 2 2
  line L35 (-61.7221, -27.7832) -> (-61.7221, -26.0315)
  line L36 (-61.7221, -26.0315) -> (-66.1879, -26.0315)
  line L37 (-57.314, -51.7293) -> (-77.6605, -51.7293)
  line L38 (-77.6605, -51.7293) -> (-77.6605, -46.1085)
  line L39 (-77.6605, -46.1085) -> (-64.3207, -46.1085)
  spline S4 degree 2 poles (-64.3207, -46.1085) (-65.3602, -44.7418) (-66.6306, -42.2009) (-67.2274, -40.276) knots 0 0 0 1 2 2 2
  line L40 (-67.2274, -40.276) -> (-62.6653, -40.276)
  spline S5 degree 2 poles (-62.6653, -40.276) (-61.7606, -43.1056) (-59.2004, -46.2432) (-57.314, -47.1287) knots 0 0 0 1 2 2 2
  line L41 (-57.314, -47.1287) -> (-57.314, -51.7293)
  point P0 (0, 0)
  constraints: 2 other
extrude "Extrusion13" cut sketch "Sketch17" against normal blind 1
chamfer "Chamfer5" distance 2 angle 45 1 edges at (-3.2876, 30.625, 6)
chamfer "Chamfer6" distance 2 angle 45 1 edges at (-78.0876, 30.625, 6)
ref_plane "Work Plane2" through (0, 0, -21) normal (0, 0, -1) x (-1, 0, 0)
chamfer "Chamfer7" distance 0.6 angle 45 24 edges at (-51.01, 47.625, 6) (-49.635, 50.0066, 6) (-46.885, 50.0066, 6) (-45.51, 47.625, 6) (-46.885, 45.2434, 6) (-49.635, 45.2434, 6) (46.885, 45.2434, 6) (45.51, 47.625, 6) (46.885, 50.0066, 6) (49.635, 50.0066, 6) (51.01, 47.625, 6) (49.635, 45.2434, 6) (46.885, -45.2434, 6) (45.51, -47.625, 6) (46.885, -50.0066, 6) (49.635, -50.0066, 6) (51.01, -47.625, 6) (49.635, -45.2434, 6) (-49.635, -50.0066, 6) (-51.01, -47.625, 6) (-49.635, -45.2434, 6) (-46.885, -45.2434, 6) (-45.51, -47.625, 6) (-46.885, -50.0066, 6)
chamfer "Chamfer8" distance 0.25 angle 45 229 edges at (-18, -62.625, 6) (57.3311, -59.6961, 6) (60.26, 4.5, 6) (-86.26, -0.5, 6) (-13, 61.625, 6) (-39.4, 23.1074, 6) (-39.5172, 1.3172, 6) (-40.9, 1.2, 6) (-42.2828, 1.3172, 6) (-42.4, 23.1074, 6) (-42.2828, 44.8976, 6) (-40.9, 45.0147, 6) (-39.5172, 44.8976, 6) (-33, 23.1074, 6) (-33.1172, 1.3172, 6) (-34.5, 1.2, 6) (-35.8828, 1.3172, 6) (-36, 23.1074, 6) (-35.8828, 44.8976, 6) (-34.5, 45.0147, 6) (-33.1172, 44.8976, 6) (-28.1, 45.0147, 6) (-26.7172, 44.8976, 6) (-26.6, 23.1074, 6) (-26.7172, 1.3172, 6) (-28.1, 1.2, 6) (-29.4828, 1.3172, 6) (-29.6, 23.1074, 6) (-29.4828, 44.8976, 6) (-21.7, 45.0147, 6) (-20.3172, 44.8976, 6) (-20.2, 23.1074, 6) (-20.3172, 1.3172, 6) (-21.7, 1.2, 6) (-23.0828, 1.3172, 6) (-23.2, 23.1074, 6) (-23.0828, 44.8976, 6) (-15.3, 45.0147, 6) (-13.9172, 44.8976, 6) (-13.8, 23.1074, 6) (-13.9172, 1.3172, 6) (-15.3, 1.2, 6) (-16.6828, 1.3172, 6) (-16.8, 23.1074, 6) (-16.6828, 44.8976, 6) (-7.4, 13.9125, 6) (-7.5172, 1.3172, 6) (-8.9, 1.2, 6) (-10.2828, 1.3172, 6) (-10.4, 13.9125, 6) (-10.2828, 26.5078, 6) (-8.9, 26.625, 6) (-7.5172, 26.5078, 6) (-1, 13.9125, 6) (-1.1172, 1.3172, 6) (-2.5, 1.2, 6) (-3.8828, 1.3172, 6) (-4, 13.9125, 6) (-3.8828, 26.5078, 6) (-2.5, 26.625, 6) (-1.1172, 26.5078, 6) (3.7, 26.625, 6) (5.0828, 26.5078, 6) (5.2, 13.9125, 6) (5.0828, 1.3172, 6) (3.7, 1.2, 6) (2.3172, 1.3172, 6) (2.2, 13.9125, 6) (2.3172, 26.5078, 6) (9.9, 45.0147, 6) (11.2828, 44.8976, 6) (11.4, 23.1074, 6) (11.2828, 1.3172, 6) (9.9, 1.2, 6) (8.5172, 1.3172, 6) (8.4, 23.1074, 6) (8.5172, 44.8976, 6) (17.6, 23.1074, 6) (17.4828, 1.3172, 6) (16.1, 1.2, 6) (14.7172, 1.3172, 6) (14.6, 23.1074, 6) (14.7172, 44.8976, 6) (16.1, 45.0147, 6) (17.4828, 44.8976, 6) (22.3, 45.0147, 6) (23.6828, 44.8976, 6) (23.8, 23.1074, 6) (23.6828, 1.3172, 6) (22.3, 1.2, 6) (20.9172, 1.3172, 6) (20.8, 23.1074, 6) (20.9172, 44.8976, 6) (29.8828, 44.8976, 6) (28.5, 45.0147, 6) (27.1172, 44.8976, 6) (27, 23.1074, 6) (27.1172, 1.3172, 6) (28.5, 1.2, 6) (29.8828, 1.3172, 6) (30, 23.1074, 6) (34.7, 45.0147, 6) (36.0828, 44.8976, 6) (36.2, 23.1074, 6) (36.0828, 1.3172, 6) (34.7, 1.2, 6) (33.3172, 1.3172, 6) (33.2, 23.1074, 6) (33.3172, 44.8976, 6) (39.4, 23.1074, 6) (39.5172, 44.8976, 6) (40.9, 45.0147, 6) (42.2828, 44.8976, 6) (42.4, 23.1074, 6) (42.2828, 1.3172, 6) (40.9, 1.2, 6) (39.5172, 1.3172, 6) (39.4, -23.0926, 6) (39.5172, -1.3172, 6) (40.9, -1.2, 6) (42.2828, -1.3172, 6) (42.4, -23.0926, 6) (42.2828, -44.8681, 6) (40.9, -44.9853, 6) (39.5172, -44.8681, 6) (34.7, -1.2, 6) (36.0828, -1.3172, 6) (36.2, -23.0926, 6) (36.0828, -44.8681, 6) (34.7, -44.9853, 6) (33.3172, -44.8681, 6) (33.2, -23.0926, 6) (33.3172, -1.3172, 6) (28.5, -1.2, 6) (29.8828, -1.3172, 6) (30, -23.0926, 6) (29.8828, -44.8681, 6) (28.5, -44.9853, 6) (27.1172, -44.8681, 6) (27, -23.0926, 6) (27.1172, -1.3172, 6) (23.8, -23.0926, 6) (23.6828, -44.8681, 6) (22.3, -44.9853, 6) (20.9172, -44.8681, 6) (20.8, -23.0926, 6) (20.9172, -1.3172, 6) (22.3, -1.2, 6) (23.6828, -1.3172, 6) (16.1, -1.2, 6) (17.4828, -1.3172, 6) (17.6, -23.0926, 6) (17.4828, -44.8681, 6) (16.1, -44.9853, 6) (14.7172, -44.8681, 6) (14.6, -23.0926, 6) (14.7172, -1.3172, 6) (9.9, -1.2, 6) (11.2828, -1.3172, 6) (11.4, -23.0926, 6) (11.2828, -44.8681, 6) (9.9, -44.9853, 6) (8.5172, -44.8681, 6) (8.4, -23.0926, 6) (8.5172, -1.3172, 6) (3.7, -1.2, 6) (5.0828, -1.3172, 6) (5.2, -23.0926, 6) (5.0828, -44.8681, 6) (3.7, -44.9853, 6) (2.3172, -44.8681, 6) (2.2, -23.0926, 6) (2.3172, -1.3172, 6) (-2.5, -1.2, 6) (-1.1172, -1.3172, 6) (-1, -23.0926, 6) (-1.1172, -44.8681, 6) (-2.5, -44.9853, 6) (-3.8828, -44.8681, 6) (-4, -23.0926, 6) (-3.8828, -1.3172, 6) (-8.9, -1.2, 6) (-7.5172, -1.3172, 6) (-7.4, -23.0926, 6) (-7.5172, -44.8681, 6) (-8.9, -44.9853, 6) (-10.2828, -44.8681, 6) (-10.4, -23.0926, 6) (-10.2828, -1.3172, 6) (-15.3, -1.2, 6) (-13.9172, -1.3172, 6) (-13.8, -23.0926, 6) (-13.9172, -44.8681, 6) (-15.3, -44.9853, 6) (-16.6828, -44.8681, 6) (-16.8, -23.0926, 6) (-16.6828, -1.3172, 6) (-23.0828, -1.3172, 6) (-23.2, -23.0926, 6) (-23.0828, -44.8681, 6) (-21.7, -44.9853, 6) (-20.3172, -44.8681, 6) (-20.2, -23.0926, 6) (-20.3172, -1.3172, 6) (-21.7, -1.2, 6) (-26.6, -23.0926, 6) (-26.7172, -44.8681, 6) (-28.1, -44.9853, 6) (-29.4828, -44.8681, 6) (-29.6, -23.0926, 6) (-29.4828, -1.3172, 6) (-28.1, -1.2, 6) (-26.7172, -1.3172, 6) (-33, -23.0926, 6) (-33.1172, -44.8681, 6) (-34.5, -44.9853, 6) (-35.8828, -44.8681, 6) (-36, -23.0926, 6) (-35.8828, -1.3172, 6) (-34.5, -1.2, 6) (-33.1172, -1.3172, 6) (-42.4, -23.0926, 6) (-42.2828, -1.3172, 6) (-40.9, -1.2, 6) (-39.5172, -1.3172, 6) (-39.4, -23.0926, 6) (-39.5172, -44.8681, 6) (-40.9, -44.9853, 6) (-42.2828, -44.8681, 6)
sketch "Sketch23" plane through (0, 0, -27) normal (0, 0, -1) x (-1, 0, 0)
  line L0 (-54.26, 34.625) -> (-60.26, 34.625) projected
  line L1 (-60.26, 34.625) -> (-60.26, -52.625) projected
  arc A0 (-60.26, -52.625) -> (-50.26, -62.625) centre (-50.26, -52.625) ccw projected
  line L2 (-50.26, -62.625) -> (86.26, -62.625) projected
  line L3 (86.26, -62.625) -> (86.26, -56.625) projected
  line L4 (86.26, -56.625) -> (-49.26, -56.625) projected
  arc A1 (-54.26, -51.625) -> (-49.26, -56.625) centre (-49.26, -51.625) ccw projected
  line L5 (-54.26, -51.625) -> (-54.26, 34.625) projected
  line L6 (-60.26, 52.625) -> (-54.26, 52.625) projected
  line L7 (-54.26, 52.625) -> (-54.26, 55.625) projected
  line L8 (-54.26, 55.625) -> (86.26, 55.625) projected
  line L9 (86.26, 55.625) -> (86.26, 61.625) projected
  line L10 (86.26, 61.625) -> (-60.26, 61.625) projected
  line L11 (-60.26, 61.625) -> (-60.26, 52.625) projected
  line L12 (-49.26, -59.625) -> (86.26, -59.625)
  line L13 (-57.26, 34.625) -> (-57.26, -51.625)
  arc A2 (-57.26, -51.625) -> (-49.26, -59.625) centre (-49.26, -51.625) ccw
  line L14 (-60.26, 52.625) -> (-54.26, 52.625) projected
  line L15 (-57.26, 52.625) -> (-57.26, 58.625)
  line L16 (-57.26, 58.625) -> (86.26, 58.625)
  line L17 (86.01, -62.375) -> (86.01, 61.375) construction
  point P0 (0, 0)
  point P1 (86.01, 58.625)
  point P2 (86.01, 55.625)
  dimension "d184" = 3
  dimension "d185" = 3
  dimension "d186" = 3
  dimension "d187" = 3
  constraints: 8 end point, 4 midpoint, 2 point on circle, 2 point on line, 1 centre point, 1 perpendicular, 1 vertical
  measures "d184" distance between parallel lines of L4 L12
  measures "d185" distance between parallel lines of L5 L13
  measures "d186" distance between parallel lines of L16 L8
  measures "d187" distance between parallel lines of L7 L15
extrude "Extrusion18" add sketch "Sketch23" along normal blind 4 contours L5 A1 L4 L3 L12 A2 L13 L0 | L15 L16 L9 L8 L7 L6
sketch "Sketch24" plane through (-86.26, -62.625, -27) normal (0, -1, 0) x (1, 0, 0)
  line L0 (136.52, 0) -> (0, 0) projected
  circle A0 centre (15, 0) radius 5
  point P0 (86.26, 27)
  dimension "d190" = 10
  dimension "d212" = 15
  constraints: 1 centre point, 1 point on line
  measures "d190" diameter of A0
  measures "d212" distance of L0.end A0.centre
extrude "Extrusion19" cut sketch "Sketch24" against normal up to surface (3 mm away)
sketch "Sketch25" plane through (60.26, -52.625, -27) normal (1, 0, 0) x (0, 0, -1)
  line L0 (0, 87.25) -> (0, 0) projected
  circle A0 centre (0, 34.25) radius 5
  line L1 (0, 114.25) -> (-32.75, 114.25) projected
  point P0 (-27, 52.625)
  point P1 (0, 29.25)
  point P2 (0, 39.25)
  dimension "d193" = 10
  dimension "d213" = 80
  constraints: 1 centre point, 1 point on line
  measures "d193" diameter of A0
  measures "d213" distance from line of L1 A0.centre
extrude "Extrusion20" cut sketch "Sketch25" against normal up to surface (3 mm away) contours L0 A0 picked at (-1.5041, 32.9541)
fillet "Fillet5" radius 2 4 edges at (58.76, -13.375, -27) (58.76, -23.375, -27) (-76.26, -61.125, -27) (-66.26, -61.125, -27)